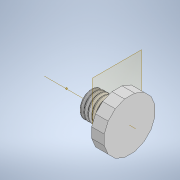
# Autodesk Inventor part: 1aThreadsV04-1_2-13-externalTest
Saved by Autodesk Inventor 2021.1 (Build 251245010, 245A)
## iProperties
Created: 2020-10-17
Part Number: 1aThreadsV04-1_2-13-externalTest
Material: Generic
Document SubType Name: Modeling
Designer: robst
Density: 1 g/cm^3
Appearance: Default
Author: robst
Autodesk Inventor part; units mm, degrees
ref_plane "XZ Plane" through (0, 0, 0) normal (0, 1, 0) x (-1, 0, 0)
ref_plane "XY Plane" through (0, 0, 0) normal (0, 0, 1) x (1, 0, 0)
sketch "ExternalTheadSketch" plane through (0, 0, 0) normal (0, 0, 1) x (1, 0, 0)
  line L0 (25.4, 6.22808) -> (29.307692, 6.22808) construction
  line L1 (29.307692, 6.22808) -> (29.307692, 5.01142) construction
  line L2 (29.307692, 5.01142) -> (25.4, 5.01142) construction
  line L3 (25.4, 5.01142) -> (25.4, 6.22808) construction
  line L4 (26.619272, 6.08816) -> (27.184469, 5.10921)
  line L5 (27.523223, 5.10921) -> (28.08842, 6.08816)
  arc A0 (27.184469, 5.10921) -> (27.523223, 5.10921) centre (27.353846, 5.207) ccw
  arc A1 (26.619272, 6.08816) -> (26.376923, 6.22808) centre (26.376923, 5.94824) ccw
  arc A2 (28.330769, 6.22808) -> (28.08842, 6.08816) centre (28.330769, 5.94824) ccw
  line L6 (26.376923, 6.22808) -> (28.330769, 6.22808)
  line L7 (26.376923, 6.22808) -> (26.376923, 5.01142) construction
  point P0 (0, 0)
  dimension "d44" = 25.4
  dimension "d45" = 6.22808
  dimension "d46" = 5.01142
  dimension "d47" = 60
  dimension "d48" = 0.19558
  dimension "d54" = 0.97692
  dimension "d55" = 1.95385
  dimension "d56" = 3.90769
  dimension "d99" = 30
  constraints: 16 end point, 7 tangent, 6 point on circle, 3 centre point, 2 parallel, 2 perpendicular, 1 equal radius, 1 horizontal, 1 point on line
  measures "d44" distance from line of L3 point (0, 0)
  measures "d45" distance from line of point (0, 0) L0
  measures "d46" distance from line of point (0, 0) L2
  measures "d47" angle of L5 L4
  measures "d48" radius of A0
  measures "d54" distance from line of A1.centre L3
  measures "d55" distance of A2.centre A1.centre
  measures "d56" distance between parallel lines of L1 L3
  measures "d99" angle of L4 L7
ref_plane "Work Plane1" through (25.4, 0, 0) normal (1, 0, 0) x (0, 1, 0)
sketch "Sketch3" plane through (25.4, 0, 0) normal (1, 0, 0) x (0, 1, 0)
  circle A0 centre (0, 0) radius 6.22808
  dimension "d81" = 12.45616
  constraints: 1 centre point, 1 coincident
  measures "d81" diameter of A0
extrude "Extrusion1" add sketch "Sketch3" against normal blind 12.7
coil "Coil1" sketch "ExternalTheadSketch" operation cut axis through (-10, 0, 0) along (-1, 0, 0) pitch 1.953846 turns 8.5 hand right
sketch "Sketch4" plane through (25.4, 0, 0) normal (1, 0, 0) x (0, 1, 0)
  line L0 (2.526187, -12.7) -> (-2.526187, -12.7)
  line L1 (-2.526187, -12.7) -> (-7.193972, -10.76654)
  line L2 (-7.193972, -10.76654) -> (-10.76654, -7.193972)
  line L3 (-10.76654, -7.193972) -> (-12.7, -2.526187)
  line L4 (-12.7, -2.526187) -> (-12.7, 2.526187)
  line L5 (-12.7, 2.526187) -> (-10.76654, 7.193972)
  line L6 (-10.76654, 7.193972) -> (-7.193972, 10.76654)
  line L7 (-7.193972, 10.76654) -> (-2.526187, 12.7)
  line L8 (-2.526187, 12.7) -> (2.526187, 12.7)
  line L9 (2.526187, 12.7) -> (7.193972, 10.76654)
  line L10 (7.193972, 10.76654) -> (10.76654, 7.193972)
  line L11 (10.76654, 7.193972) -> (12.7, 2.526187)
  line L12 (12.7, 2.526187) -> (12.7, -2.526187)
  line L13 (12.7, -2.526187) -> (10.76654, -7.193972)
  line L14 (10.76654, -7.193972) -> (7.193972, -10.76654)
  line L15 (7.193972, -10.76654) -> (2.526187, -12.7)
  point P0 (0, 0)
  point P1 (0, 0)
  dimension "d93" = 25.4
  constraints: 32 end point, 1 coincident, 1 horizontal, 33 other
  measures "d93" distance between parallel lines of L8 L0
extrude "Extrusion2" add sketch "Sketch4" along normal blind 6.35
equation "\"d45\" = a1MajorRadius"
equation "\"d46\" = a1MinorRadius"
equation "\"d47\" = threadAngle"
equation "\"d48\" = a1RootRadius"
equation "\"d54\" = 0.5 * pitch"
equation "\"d55\" = pitch"
equation "\"d56\" = 2 * pitch"
equation "\"d99\" = 0.5 * threadAngle"
equation "\"d81\" = a1MajorDiameter"
equation "\"d85\" = pitch"
equation "\"threadAngle\" = 60deg"
equation "\"a1MajorDiameter\" = 12.45616"
equation "\"a1MajorRadius\" = 0.5 * a1MajorDiameter"
equation "\"a1MinorDiameter\" = 10.02284"
equation "\"a1MinorRadius\" = 0.5 * a1MinorDiameter"
equation "\"a1RootRadius\" = 0.19558"
equation "\"a1CrestRadiusMax\" = 0.21082"
equation "\"a1ThreadDepth\" = 1.21666"
equation "\"pitch\" = 1.953846"
body "Solid1"
